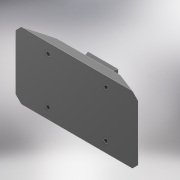
# Autodesk Inventor part: 2
Saved by Autodesk Inventor 2022 (Build 260153000, 153)
## iProperties
Company: HS Emden/Leer
Created: 2023-12-30
Part Number: 2
Material: PMMA-Kunststoff
Document SubType Name: Modeling
Designer: Yaman Alsaady
Density: 1.188 g/cm^3
Appearance: Glatt - Schwarz
Project: Delta-Robot
Author: Yaman Alsaady
Title: Base
## iProperties of the stored document 5,1_3D-Druck.ipt
Created: 2023-12-30
Part Number: 5,1_3D-Druck
Material: Generisch
Document SubType Name: Modeling
Designer: alsaa
Density: 1 g/cm^3
Appearance: Vorgabe
Author: alsaa
Autodesk Inventor part; units mm, degrees
ref_plane "YZ Plane" through (0, 0, 0) normal (1, 0, 0) x (0, 1, 0)
ref_plane "XZ Plane" through (0, 0, 0) normal (0, 1, 0) x (-1, 0, 0)
ref_plane "Arbeitsebene1" through (0, 0, 10) normal (0, 0, 1) x (1, 0, 0)
sketch "Skizze1" plane through (0, 0, 0) normal (0, 0, 1) x (1, 0, 0)
  line L0 (-27.5, 25.5) -> (27.5, 25.5)
  line L1 (32.5, 20.5) -> (32.5, -20.5)
  line L2 (27.5, -25.5) -> (-27.5, -25.5)
  line L3 (-32.5, -20.5) -> (-32.5, 20.5)
  line L4 (-32.5, 0) -> (32.5, 0) construction
  line L5 (0, 25.5) -> (0, -25.5) construction
  line L6 (-32.5, 20.5) -> (-27.5, 25.5)
  line L7 (32.5, 20.5) -> (27.5, 25.5)
  line L8 (-32.5, -20.5) -> (-27.5, -25.5)
  line L9 (32.5, -20.5) -> (27.5, -25.5)
  point P0 (0, 0)
  point P1 (0, 0)
  dimension "d0" = 65
  dimension "d3" = 5
  dimension "d4" = 51
  dimension "d28" = 5
  constraints: 20 end point, 6 symmetric about line, 5 midpoint, 4 parallel, 1 coincident, 1 horizontal, 1 perpendicular
  measures "d0" distance of L4.start L4.end
  measures "d3" distance from line of L0.start L3
  measures "d4" distance of L5.start L5.end
  measures "d28" distance from line of L0 L3.end
sketch "Skizze2" plane through (0, 0, 10) normal (0, 0, 1) x (1, 0, 0)
  line L0 (-48, 29) -> (48, 29)
  line L1 (53, 24) -> (53, -24)
  line L2 (48, -29) -> (-48, -29)
  line L3 (-53, -24) -> (-53, 24)
  line L4 (-53, 0) -> (53, 0) construction
  line L5 (0, 29) -> (0, -29) construction
  line L6 (-53, 24) -> (-48, 29)
  line L7 (53, 24) -> (48, 29)
  line L8 (-53, -24) -> (-48, -29)
  line L9 (53, -24) -> (48, -29)
  point P0 (0, 0)
  point P1 (0, 0)
  dimension "d6" = 58
  dimension "d8" = 45
  dimension "d9" = 5
  dimension "d10" = 106
  constraints: 20 end point, 6 symmetric about line, 5 midpoint, 2 parallel, 1 coincident, 1 horizontal, 1 perpendicular
  measures "d6" distance of L5.start L5.end
  measures "d8" angle of L4 L6
  measures "d9" distance from line of L0.start L3
  measures "d10" distance of L4.start L4.end
loft "Erhebung1" add profiles "Skizze1", "Skizze2"
sketch "Skizze3" plane through (27.5, 25.5, 0) normal (0, 0, -1) x (-1, 0, 0)
  line L0 (14, -51) -> (41, -51)
  line L1 (41, -51) -> (41, -9)
  line L2 (41, -9) -> (14, -9)
  line L3 (14, -9) -> (14, -51)
  line L4 (55, -51) -> (0, -51) projected
  point P0 (27.5, -25.5)
  point P1 (27.5, -51)
  dimension "d15" = 27
  dimension "d16" = 42
  constraints: 8 end point, 2 midpoint, 2 parallel, 1 horizontal, 1 perpendicular
  measures "d15" distance between parallel lines of L1 L3
  measures "d16" distance of L0.end L1.end
extrude "Extrusion1" add sketch "Skizze3" along normal blind 13
sketch "Skizze4" plane through (-13.5, -25.5, 0) normal (0, -1, 0) x (1, 0, 0)
  line L0 (13.5, 0) -> (13.5, -13) construction
  line L1 (27, -13) -> (0, -13) construction
  circle A0 centre (13.5, -6.5) radius 2.15
  line L2 (27, 0) -> (27, -13) projected
  line L3 (27, -13) -> (22.5, 0)
  line L4 (0, 0) -> (27, 0) projected
  line L5 (0, -13) -> (4.5, 0)
  line L6 (0, 0) -> (27, 0) projected
  line L7 (0, 0) -> (0, -13) projected
  line L8 (27, -13) -> (0, -13) projected
  line L9 (27, 0) -> (27, -13) projected
  line L10 (26.6825, -13) -> (22.1825, 0)
  line L11 (4.8175, 0) -> (0.3175, -13)
  line L12 (0.1038, -12.7) -> (26.8962, -12.7)
  point P0 (26.5787, -12.7)
  point P1 (0.4213, -12.7)
  point P2 (22.1825, 0)
  dimension "d19" = 18
  dimension "d20" = 4.3
  dimension "d29" = 27
  dimension "d30" = 13
  dimension "d31" = 0.3
  dimension "d32" = 0.3
  dimension "d33" = 0.3
  constraints: 12 end point, 8 point on line, 2 midpoint, 2 parallel, 1 centre point, 1 horizontal, 1 other
  measures "d19" distance of L5.end L3.end
  measures "d20" diameter of A0
  measures "d29" distance of L1.end L1.start
  measures "d30" distance of L2.start L1.start
  measures "d31" distance between parallel lines of L5 L11
  measures "d32" distance between parallel lines of L10 L3
  measures "d33" distance between parallel lines of L12 L1
extrude "Extrusion2" cut sketch "Skizze4" against normal through all contours A0 | L2 L3 L4 | L8 L10 L12 L3 | L3 L12 L10 L4 | L8 L11 L12 L10 | L8 L5 L12 L11 | L11 L12 L5 L4 | L7 L4 L5
sketch "Skizze5" plane through (27.5, 25.5, 0) normal (0, 0, -1) x (-1, 0, 0)
  line L0 (2.5, -5.5) -> (52.5, -5.5)
  line L1 (52.5, -5.5) -> (52.5, -45.5)
  line L2 (52.5, -45.5) -> (2.5, -45.5)
  line L3 (2.5, -45.5) -> (2.5, -5.5)
  line L4 (2.5, -5.5) -> (52.5, -45.5) construction
  line L5 (52.5, -5.5) -> (2.5, -45.5) construction
  circle A0 centre (2.5, -5.5) radius 1.75
  circle A1 centre (52.5, -5.5) radius 1.75
  circle A2 centre (2.5, -45.5) radius 1.75
  circle A3 centre (52.5, -45.5) radius 1.75
  point P0 (27.5, -25.5)
  point P1 (27.5, -25.5)
  point P2 (27.5, -25.5)
  dimension "d23" = 50
  dimension "d24" = 40
  dimension "d25" = 3.5
  constraints: 12 end point, 5 coincident, 4 centre point, 3 equal radius, 3 midpoint, 2 parallel, 1 horizontal, 1 perpendicular
  measures "d23" distance of L0.start L0.end
  measures "d24" distance of L0.end L1.end
  measures "d25" diameter of A0
extrude "Extrusion3" cut sketch "Skizze5" against normal through all contours L3 A0 L0 | L0 A0 L3 | A1 L1 L0 | L0 L1 A1 | A2 L2 L3 | L3 L2 A2 | A3 L2 L1 | L1 L2 A3
sketch "Skizze6" plane through (27.5, 25.5, 0) normal (0, 0, -1) x (-1, 0, 0)
  circle A0 centre (2.5, -5.5) radius 1.75 projected
  line L0 (-0.9641, -5.5) -> (0.7679, -2.5)
  line L1 (0.7679, -2.5) -> (4.2321, -2.5)
  line L2 (4.2321, -2.5) -> (5.9641, -5.5)
  line L3 (5.9641, -5.5) -> (4.2321, -8.5)
  line L4 (4.2321, -8.5) -> (0.7679, -8.5)
  line L5 (0.7679, -8.5) -> (-0.9641, -5.5)
  line L6 (0, 0) -> (55, 0) projected
  line L7 (27.5, 0) -> (27.5, -51) construction
  line L8 (36.1825, -51) -> (18.8175, -51) construction
  line L9 (-5, -46) -> (-5, -5) construction
  line L10 (-5, -25.5) -> (60, -25.5) construction
  line L11 (60, -5) -> (60, -46) construction
  circle A1 centre (52.5, -5.5) radius 1.75
  line L12 (55.9641, -5.5) -> (54.2321, -2.5)
  line L13 (54.2321, -2.5) -> (50.7679, -2.5)
  line L14 (50.7679, -2.5) -> (49.0359, -5.5)
  line L15 (49.0359, -5.5) -> (50.7679, -8.5)
  line L16 (50.7679, -8.5) -> (54.2321, -8.5)
  line L17 (54.2321, -8.5) -> (55.9641, -5.5)
  line L18 (55, 0) -> (0, 0)
  circle A2 centre (2.5, -45.5) radius 1.75
  line L19 (-0.9641, -45.5) -> (0.7679, -48.5)
  line L20 (0.7679, -48.5) -> (4.2321, -48.5)
  line L21 (4.2321, -48.5) -> (5.9641, -45.5)
  line L22 (5.9641, -45.5) -> (4.2321, -42.5)
  line L23 (4.2321, -42.5) -> (0.7679, -42.5)
  line L24 (0.7679, -42.5) -> (-0.9641, -45.5)
  line L25 (54.2321, -48.5) -> (50.7679, -48.5)
  line L26 (55.9641, -45.5) -> (54.2321, -48.5)
  circle A3 centre (52.5, -45.5) radius 1.75
  line L27 (50.7679, -48.5) -> (49.0359, -45.5)
  line L28 (54.2321, -42.5) -> (55.9641, -45.5)
  line L29 (50.7679, -42.5) -> (54.2321, -42.5)
  line L30 (49.0359, -45.5) -> (50.7679, -42.5)
  point P0 (27.5, -25.5)
  dimension "d34" = 6
  constraints: 54 end point, 26 symmetric about line, 4 coincident, 4 midpoint, 3 centre point, 1 parallel, 16 other
  measures "d34" distance between parallel lines of L4 L1
extrude "Extrusion4" cut sketch "Skizze6" against normal blind 6 contours A0 | L0 L1 L2 L3 L4 L5 | A1 | L17 L16 L15 L14 L13 L12 | A2 | L24 L23 L22 L21 L20 L19 | L25 L27 L30 L29 L28 L26 | A3
sketch "Skizze7" plane through (-8.6825, 16.5, 0) normal (0, 1, 0) x (1, 0, 0)
  circle A0 centre (8.6825, 6.5) radius 2.15 projected
  line L0 (6.5752, 10.15) -> (10.7899, 10.15)
  line L1 (10.7899, 10.15) -> (12.8972, 6.5)
  line L2 (12.8972, 6.5) -> (10.7899, 2.85)
  line L3 (10.7899, 2.85) -> (6.5752, 2.85)
  line L4 (6.5752, 2.85) -> (4.4679, 6.5)
  line L5 (4.4679, 6.5) -> (6.5752, 10.15)
  line L6 (21.7612, 12.7) -> (-4.3962, 12.7) projected
  line L7 (4.4679, 6.5) -> (4.4679, 12.7)
  line L8 (12.8972, 6.5) -> (12.8972, 12.7)
  line L9 (-4.3962, 12.7) -> (21.7612, 12.7) projected
  line L10 (4.4679, 12.7) -> (12.8972, 12.7)
  point P0 (8.6825, 0)
  dimension "d37" = 7.3
  constraints: 18 end point, 2 point on line, 1 coincident, 1 collinear, 1 parallel, 1 perpendicular, 1 vertical, 13 other
  measures "d37" distance between parallel lines of L3 L0
extrude "Extrusion5" cut sketch "Skizze7" against normal blind 10
extrude "Extrusion6" add sketch "Skizze7" against normal blind 6.5
equation "\"d32\" = d31"
equation "\"d33\" = d32"
